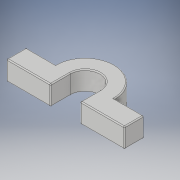
# Autodesk Inventor part: Motor hoop
Saved by Autodesk Inventor 2019 (Build 230136000, 136)
## iProperties
Created: 2021-03-23
Part Number: Motor hoop
Material: Generic
Document SubType Name: Modeling
Designer: User
Density: 1 g/cm^3
Appearance: Default
Author: User
Autodesk Inventor part; units mm, degrees
ref_plane "YZ Plane" through (0, 0, 0) normal (1, 0, 0) x (0, 1, 0)
ref_plane "XZ Plane" through (0, 0, 0) normal (0, 1, 0) x (-1, 0, 0)
ref_plane "XY Plane" through (0, 0, 0) normal (0, 0, 1) x (1, 0, 0)
sketch "Sketch1" plane through (0, 0, 0) normal (0, 1, 0) x (-1, 0, 0)
  arc A0 (-15, 0) -> (15, 0) centre (0, 0) ccw
  arc A1 (-7.5, 0) -> (7.5, 0) centre (0, 0) ccw
  line L0 (-30, 0) -> (-30, 10)
  line L1 (30, 10) -> (30, 0)
  line L2 (-30, 0) -> (-15, 0)
  line L3 (15, 0) -> (30, 0)
  line L4 (7.5, 0) -> (7.5, 10)
  line L5 (-7.5, 0) -> (-7.5, 10)
  line L6 (-30, 10) -> (-7.5, 10)
  line L7 (7.5, 10) -> (30, 10)
  dimension "d0" = 30
  dimension "d1" = 15
  dimension "d6" = 10
  dimension "d7" = 15
  dimension "d9" = 10
  dimension "d10" = 0
  dimension "d11" = 30
  dimension "d12" = 10
  dimension "d15" = 30
  dimension "d16" = 37.5
  constraints: 16 end point, 4 perpendicular, 4 point on circle, 2 centre point, 2 coincident, 2 parallel, 1 vertical
  measures "d0" diameter of A0
  measures "d1" diameter of A1
  measures "d6" distance between parallel lines of L3 L7
  measures "d7" distance between parallel lines of L5 L4
  measures "d9" distance between parallel lines of L6 L2
  measures "d10" distance between parallel lines of L7 L6
  measures "d11" distance from line of point (0, 0) L1
  measures "d12" distance from line of point (0, 0) L7
  measures "d15" distance from line of L0 point (0, 0)
  measures "d16" distance from line of L5.start L1
extrude "Extrusion1" add sketch "Sketch1" along normal mid plane 10
fillet "Fillet1" radius 0.5 23 edges at (-18.75, 5, 10) (-18.75, -5, 10) (0, 5, -7.5) (7.5, 5, 5) (-7.5, 5, 5) (-7.5, -5, 5) (7.5, -5, 5) (0, -5, -7.5) (18.75, 5, 10) (18.75, -5, 10) (22.5, 5, 0) (30, 5, 5) (30, 0, 0) (30, 0, 10) (22.5, -5, 0) (0, -5, -15) (0, 5, -15) (-22.5, 5, 0) (-30, 0, 0) (-30, 0, 10) (-30, 5, 5) (-30, -5, 5) (-7.5, 0, 10)
fillet "Fillet1" radius 0.5 26 edges at (30, 5, 5) (30, 0, 10) (30, -5, 5) (30, 0, 0) (22.5, 5, 0) (22.5, -5, 0) (18.75, 5, 10) (7.5, 0, 10) (18.75, -5, 10) (7.5, 5, 5) (0, 5, -7.5) (-7.5, 5, 5) (-18.75, 5, 10) (-30, 5, 5) (-22.5, 5, 0) (0, 5, -15) (0, -5, -15) (7.5, -5, 5) (0, -5, -7.5) (-7.5, -5, 5) (-18.75, -5, 10) (-30, -5, 5) (-22.5, -5, 0) (-7.5, 0, 10) (-30, 0, 10) (-30, 0, 0)
body "Solid1"
